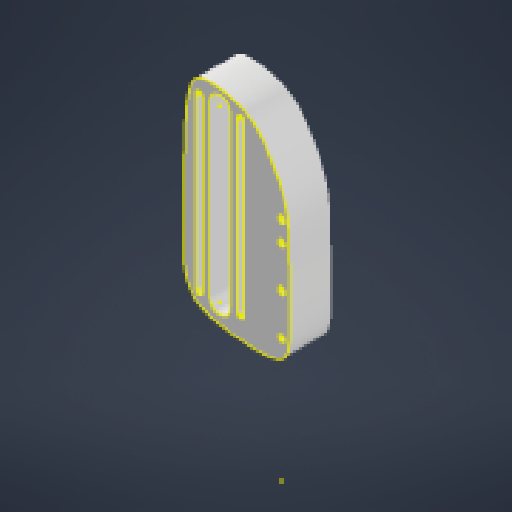
# Autodesk Inventor part: first-stage
Saved by Autodesk Inventor 2023 (Build 270158000, 158)
## iProperties
Created: 2023-03-31
Part Number: first-stage
Material: Generic
Document SubType Name: Modeling
Designer: eduar
Density: 1 g/cm^3
Appearance: Default
Author: eduar
Autodesk Inventor part; units mm, degrees
ref_plane "YZ Plane" through (0, 0, 0) normal (1, 0, 0) x (0, 1, 0)
ref_plane "XZ Plane" through (0, 0, 0) normal (0, 1, 0) x (-1, 0, 0)
ref_plane "XY Plane" through (0, 0, 0) normal (0, 0, 1) x (1, 0, 0)
sketch "Sketch1" plane through (0, 0, 0) normal (0, 0, 1) x (1, 0, 0)
  circle A0 centre (0, 139.7) radius 2.1844 projected
  circle A1 centre (0, 127) radius 2.1844 projected
  circle A2 centre (0, 101.6) radius 2.1844 projected
  circle A3 centre (0, 76.2) radius 2.0828 projected
  circle A4 centre (-38.1, 180.975) radius 6.35
  line L0 (-38.1, 180.975) -> (-38.1, 76.2)
  circle A5 centre (0, 50.8) radius 2.1844 projected
  circle A6 centre (-38.1, 76.2) radius 6.35
  line L1 (-44.45, 76.2) -> (-44.45, 180.975)
  line L2 (-31.75, 180.975) -> (-31.75, 76.2)
  line L3 (-38.1, 180.975) -> (-50.8, 180.975)
  line L4 (-38.1, 180.975) -> (-25.4, 180.975)
  circle A7 centre (-25.4, 180.975) radius 2.0955
  circle A8 centre (-50.8, 180.975) radius 2.0955
  line L5 (-38.1, 76.2) -> (-50.8, 76.2)
  line L6 (-38.1, 76.2) -> (-25.4, 76.2)
  circle A9 centre (-25.4, 76.2) radius 2.0574
  circle A10 centre (-50.8, 76.2) radius 2.0574
  line L7 (-52.8574, 76.1993) -> (-52.8955, 180.9742)
  line L8 (-23.3426, 76.1993) -> (-23.3045, 180.9742)
  line L9 (-27.4574, 76.2) -> (-27.4955, 180.975)
  line L10 (-48.7426, 76.2) -> (-48.7045, 180.975)
  line L11 (-60.325, 87.3125) -> (-58.7375, 74.1426) construction
  line L12 (-58.7375, 74.1426) -> (-50.8, 65.0875) construction
  line L13 (-50.8, 65.0875) -> (-22.225, 61.9125) construction
  line L14 (-22.225, 61.9125) -> (0, 61.9125) construction
  line L15 (0, 61.9125) -> (6.35, 69.85) construction
  line L16 (6.35, 69.85) -> (4.7625, 103.7844) construction
  line L17 (4.7625, 103.7844) -> (4.7625, 128.5875) construction
  line L18 (4.7625, 128.5875) -> (4.7625, 149.225) construction
  line L19 (4.7625, 149.225) -> (-9.525, 174.625) construction
  line L20 (-9.525, 174.625) -> (-20.6375, 188.9125) construction
  line L21 (-20.6375, 188.9125) -> (-47.625, 192.0875) construction
  line L22 (-47.625, 192.0875) -> (-60.325, 192.0875) construction
  line L23 (-60.325, 192.0875) -> (-60.325, 149.225) construction
  line L24 (-60.325, 149.225) -> (-60.325, 87.3125) construction
  spline S0 degree 4 poles (-60.325, 87.3125) (-58.7375, 74.1426) (-50.8, 65.0875) (-22.225, 61.9125) (0, 61.9125) (6.35, 69.85) (4.7625, 103.7844) (4.7625, 128.5875) (4.7625, 149.225) (-9.525, 174.625) (-20.6375, 188.9125) (-47.625, 192.0875) (-60.325, 192.0875) (-60.325, 149.225) (-60.325, 87.3125) knots 1 1 1 1 1 2 3 4 5 6 7 8 9 10 11 12 12 12 12 12
  point P0 (0, 0)
  point P1 (-23.3426, 76.2)
  dimension "d2" = 12.7
  dimension "d4" = 25.4
  dimension "d5" = 12.7
  dimension "d6" = 12.7
  dimension "d8" = 4.191
  dimension "d9" = 4.191
  dimension "d10" = 12.7
  dimension "d11" = 4.1148
  dimension "d12" = 4.1148
  dimension "d13" = 12.7
  dimension "d14" = 12.7
  constraints: 22 end point, 12 point on circle, 8 tangent, 6 centre point, 6 horizontal, 5 coincident, 5 vertical, 4 point on line, 3 other
  measures "d2" diameter of A4
  measures "d4" vertical distance of A5.centre L0.end
  measures "d5" diameter of A6
  measures "d6" distance of L0.start L3.end
  measures "d8" diameter of A7
  measures "d9" diameter of A8
  measures "d10" distance of L0.start L4.end
  measures "d11" diameter of A9
  measures "d12" diameter of A10
  measures "d13" distance of L5.start L6.end
  measures "d14" distance of L5.start L5.end
extrude "Extrusion1" add sketch "Sketch1" along normal blind 25.4 contours L4 L9 L6 L2 | L1 L5 L10 L3 | S0
sketch "Sketch2" plane through (0, 0, 25.4) normal (0, 0, 1) x (1, 0, 0)
  arc A0 (-23.3045, 180.9742) -> (-27.4955, 180.975) centre (-25.4, 180.975) ccw projected
  line L0 (-23.3045, 180.9742) -> (-23.3426, 76.2) projected
  arc A1 (-27.4574, 76.2) -> (-23.3426, 76.2) centre (-25.4, 76.2) ccw projected
  line L1 (-27.4574, 76.2) -> (-27.4955, 180.975) projected
  line L2 (-31.75, 180.975) -> (-31.75, 76.2) projected
  arc A2 (-44.45, 76.2) -> (-31.75, 76.2) centre (-38.1, 76.2) ccw projected
  line L3 (-44.45, 76.2) -> (-44.45, 180.975) projected
  arc A3 (-31.75, 180.975) -> (-44.45, 180.975) centre (-38.1, 180.975) ccw projected
  line L4 (-48.7045, 180.975) -> (-48.7426, 76.2) projected
  arc A4 (-52.8574, 76.1993) -> (-48.7426, 76.2) centre (-50.8, 76.2) ccw projected
  line L5 (-52.8574, 76.1993) -> (-52.8955, 180.9742) projected
  arc A5 (-48.7045, 180.975) -> (-52.8955, 180.9742) centre (-50.8, 180.975) ccw projected
  circle A6 centre (0, 76.2) radius 2.0828 projected
  circle A7 centre (0, 101.6) radius 2.1844 projected
  circle A8 centre (0, 127) radius 2.1844 projected
  circle A9 centre (0, 139.7) radius 2.1844 projected
  point P0 (0, 0)
  constraints: 1 other
body "Solid1"
